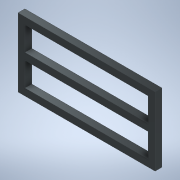
# Autodesk Inventor part: Base_mesa
Saved by Autodesk Inventor 2020 (Build 240168000, 168)
## iProperties
Created: 2020-07-18
Part Number: Base_mesa
Material: Hierro, fundido
Document SubType Name: Modeling
Designer: louis
Density: 7.15 g/cm^3
Appearance: Gris hierro
Author: louis
Autodesk Inventor part; units mm, degrees
ref_plane "YZ Plane" through (0, 0, 0) normal (1, 0, 0) x (0, 1, 0)
ref_plane "XZ Plane" through (0, 0, 0) normal (0, 1, 0) x (-1, 0, 0)
ref_plane "XY Plane" through (0, 0, 0) normal (0, 0, 1) x (1, 0, 0)
sketch "Boceto1" plane through (0, 0, 0) normal (0, 0, 1) x (1, 0, 0)
  line L0 (-508.547, 495.7265) -> (491.453, 495.7265)
  line L1 (491.453, 495.7265) -> (491.453, -4.2735)
  line L2 (491.453, -4.2735) -> (-508.547, -4.2735)
  line L3 (-508.547, -4.2735) -> (-508.547, 495.7265)
  line L4 (-458.547, 445.7265) -> (441.453, 445.7265)
  line L5 (441.453, 45.7265) -> (-458.547, 45.7265)
  line L6 (441.453, 270.7265) -> (-458.547, 270.7265)
  line L7 (-458.547, 220.7265) -> (441.453, 220.7265)
  line L8 (-458.547, 270.7265) -> (-458.547, 445.7265)
  line L9 (-458.547, 220.7265) -> (-458.547, 45.7265)
  line L10 (441.453, 270.7265) -> (441.453, 445.7265)
  line L11 (441.453, 220.7265) -> (441.453, 45.7265)
  point P0 (0, 0)
  dimension "d0" = 1000
  dimension "d1" = 500
  dimension "d2" = 900
  dimension "d4" = 400
  dimension "d5" = 50
  dimension "d17" = 175
  dimension "d18" = 175
  dimension "d19" = 175
  dimension "d20" = 175
  constraints: 24 end point, 5 equal length, 2 horizontal, 2 perpendicular, 1 vertical
  measures "d0" distance of L0.start L0.end
  measures "d1" distance of L0.end L1.end
  measures "d2" distance of L4.start L4.end
  measures "d4" distance of L5.end L4.start
  measures "d5" distance between parallel lines of L2 L5
  measures "d17" distance of L7.start L5.end
  measures "d18" distance of L7.end L5.start
  measures "d19" distance of L6.end L4.start
  measures "d20" distance of L6.start L4.end
extrude "Extrusión1" add sketch "Boceto1" along normal blind 50
